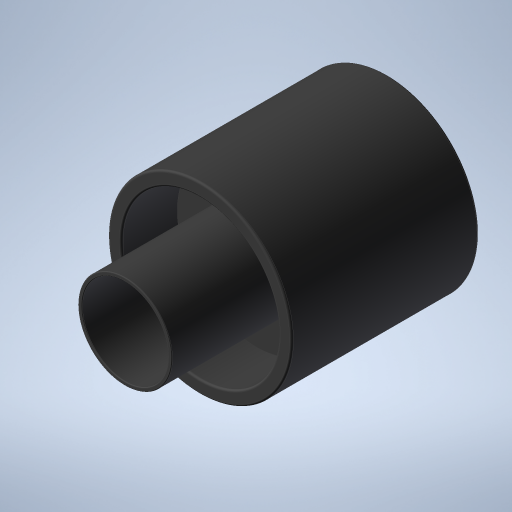
# Autodesk Inventor part: Part4
Saved by Autodesk Inventor 2024 (Build 280153000, 153)
## iProperties
Created: 2024-06-14
Part Number: Part4
Material: Generic
Document SubType Name: Sheet Metal
Designer: albah
Density: 1 g/cm^3
Sheet Metal Rule: Default_mm
Appearance: Default
Author: albah
Autodesk Inventor part; units mm, degrees
ref_plane "YZ Plane" through (0, 0, 0) normal (1, 0, 0) x (0, 1, 0)
ref_plane "XZ Plane" through (0, 0, 0) normal (0, 1, 0) x (-1, 0, 0)
ref_plane "XY Plane" through (0, 0, 0) normal (0, 0, 1) x (1, 0, 0)
sketch "Sketch1" plane through (0, 0, 0) normal (0, 0, 1) x (1, 0, 0)
  circle A0 centre (0, 0) radius 12.5
  circle A1 centre (0, 0) radius 11.5
  circle A2 centre (0, 0) radius 24.5
  circle A3 centre (0, 0) radius 21
  dimension "d0" = 25
  dimension "d1" = 23
  dimension "d2" = 49
  dimension "d3" = 42
  constraints: 4 centre point, 4 coincident
  measures "d0" diameter of A0
  measures "d1" diameter of A1
  measures "d2" diameter of A2
  measures "d3" diameter of A3
extrude "Extrusion1" add sketch "Sketch1" along normal blind 40 contours A0
extrude "Extrusion2" add sketch "Sketch1" along normal blind 20 contours A2
extrude "Extrusion3" add sketch "Sketch1" along normal blind 5 contours A3
fillet "Fillet1" radius 0.5 2 edges at (-21, 0, 20) (-24.5, 0, 20)
sketch "Sketch2" plane through (0, 0, 0) normal (0, 0, -1) x (-1, 0, 0)
  circle A0 centre (0, 0) radius 24.5
  circle A1 centre (0, 0) radius 22.5
  dimension "d11" = 49
  dimension "d12" = 45
  constraints: 2 centre point, 2 coincident
  measures "d11" diameter of A0
  measures "d12" diameter of A1
extrude "Extrusion4" add sketch "Sketch2" along normal blind 30
fillet "Fillet2" radius 0.5 2 edges at (24.5, 0, -30) (22.5, 0, -30)
fillet "Fillet3" radius 0.2 2 edges at (-12.5, 0, 40) (-11.5, 0, 40)
equation "\"BendRadius\" = Thickness"
equation "\"BendReliefWidth\" = Thickness"
equation "\"BendReliefDepth\" = 0.5 * Thickness"
equation "\"CornerReliefSize\" = 4 * Thickness"
equation "\"MinimumRemnant\" = 2 * Thickness"
equation "\"TransitionRadius\" = BendRadius"
equation "\"JacobiRadiusSize\" = BendRadius"
equation "\"GapSize\" = Thickness"
equation "\"Thickness\" = 0.5"
body "Solid1"
